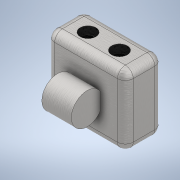
# Autodesk Inventor part: Camera2
Saved by Autodesk Inventor 2022 (Build 260153000, 153)
## iProperties
Created: 2021-10-29
Part Number: Camera2
Material: Generic
Document SubType Name: Modeling
Designer: Mark Maara
Density: 1 g/cm^3
Appearance: Satin Brushed
Author: Mark Maara
Autodesk Inventor part; units mm, degrees
ref_plane "YZ Plane" through (0, 0, 0) normal (1, 0, 0) x (0, 1, 0)
ref_plane "XZ Plane" through (0, 0, 0) normal (0, 1, 0) x (-1, 0, 0)
ref_plane "XY Plane" through (0, 0, 0) normal (0, 0, 1) x (1, 0, 0)
sketch "Sketch1" plane through (0, 0, 0) normal (1, 0, 0) x (0, 1, 0)
  circle A0 centre (0, 0) radius 40
  dimension "d0" = 80
  constraints: 1 centre point, 1 coincident
  measures "d0" diameter of A0
extrude "Extrusion1" add sketch "Sketch1" along normal blind 75
ref_plane "Work Plane1" through (37.5, 0, 0) normal (1, 0, 0) x (0, 0, -1)
sketch "Sketch2" plane through (37.5, 0, 0) normal (1, 0, 0) x (0, 0, -1)
  line L0 (0, 0) -> (35, 0)
  line L1 (35, 0) -> (130, 0)
  line L2 (130, 0) -> (130, 90)
  line L3 (130, 90) -> (35, 90)
  line L4 (35, 90) -> (35, 0)
  line L5 (130, 0) -> (130, -90)
  line L6 (130, -90) -> (35, -90)
  line L7 (35, -90) -> (35, 0)
  dimension "d3" = 35
  dimension "d6" = 90
  dimension "d9" = 95
  constraints: 16 end point, 2 horizontal, 2 parallel, 2 symmetric about line, 1 perpendicular
  measures "d3" distance of L0.start L0.end
  measures "d6" distance of L1.end L2.end
  measures "d9" distance of L5.end L7.start
extrude "Extrusion2" add sketch "Sketch2" along normal mid plane 200
fillet "Fillet1" radius 20 8 edges at (137.5, 90, -82.5) (37.5, 90, -130) (137.5, 0, -130) (137.5, -90, -82.5) (37.5, -90, -130) (-62.5, 0, -130) (-62.5, 90, -82.5) (-62.5, -90, -82.5)
fillet "Fillet2" radius 20 8 edges at (131.6421, -84.1421, -35) (137.5, 0, -35) (131.6421, 84.1421, -35) (37.5, 90, -35) (-56.6421, 84.1421, -35) (-62.5, 0, -35) (-56.6421, -84.1421, -35) (37.5, -90, -35)
sketch "Sketch3" plane through (-42.5, 90, -110) normal (0, 1, 0) x (1, 0, 0)
  line L0 (160, 0) -> (180, 0) projected
  line L1 (0, 0) -> (160, 0)
  line L2 (160, 0) -> (80, 0)
  line L3 (160, 0) -> (0, 0) projected
  line L4 (80, 0) -> (80, -30)
  line L5 (80, -30) -> (120, -30)
  circle A0 centre (120, -30) radius 20
  circle A1 centre (40, -30) radius 20
  point P0 (42.5, -110)
  dimension "d10" = 30
  dimension "d11" = 40
  constraints: 8 end point, 2 centre point, 2 horizontal, 1 coincident, 1 midpoint, 1 symmetric about line, 1 vertical, 1 other
  measures "d10" distance of L2.end L4.end
  measures "d11" diameter of A0
extrude "Extrusion3" cut sketch "Sketch3" against normal blind 20
body "Solid1"
